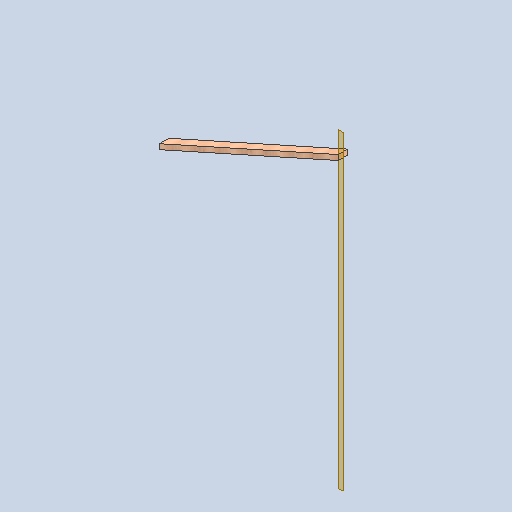
# Autodesk Inventor part: back slant
Saved by Autodesk Inventor 2025 (Build 290162000, 162)
## iProperties
Created: 2024-09-05
Part Number: back slant
Material: Wood (Birch)
Document SubType Name: Modeling
Designer: Win
Density: 0.55 g/cm^3
Appearance: Birch - Natural Polished
Author: Win
Autodesk Inventor part; units mm, degrees
ref_plane "YZ Plane" through (0, 0, 0) normal (1, 0, 0) x (0, 1, 0)
ref_plane "XZ Plane" through (0, 0, 0) normal (0, 1, 0) x (-1, 0, 0)
ref_plane "XY Plane" through (0, 0, 0) normal (0, 0, 1) x (1, 0, 0)
ref_plane "Work Plane1" through (0, 81.2927, 0) normal (0, 0, 1) x (1, 0, 0)
ref_plane "Work Plane2" through (0, 81.2927, 0) normal (0, 0, 1) x (1, 0, 0)
sketch "Sketch2" plane through (0, 81.2927, 0) normal (0, 0, 1) x (1, 0, 0)
  line L0 (-1930.4, 883.9073) -> (-1879.6, 883.9073) projected
  line L1 (-1879.6, 2103.1073) -> (-1879.6, 883.9073) projected
  line L2 (-1930.4, 2103.1073) -> (-1879.6, 2103.1073) projected
  line L3 (-1930.4, 2103.1073) -> (-1930.4, 883.9073) projected
  line L4 (-50.8, 2001.5073) -> (-50.8, 2103.1073) projected
  line L5 (-50.8, 2103.1073) -> (-1879.6, 2103.1073) projected
  line L6 (-1879.6, 2001.5073) -> (-1879.6, 2103.1073) projected
  line L7 (-50.8, 2001.5073) -> (-1879.6, 2001.5073) projected
  line L8 (0, -81.2927) -> (50.8, -81.2927) projected
  line L9 (50.8, -81.2927) -> (50.8, 2966.7073) projected
  line L10 (0, 2966.7073) -> (50.8, 2966.7073) projected
  line L11 (0, -81.2927) -> (0, 2966.7073) projected
  line L12 (-1930.4, 2103.1073) -> (0, 2966.7073)
  line L13 (0, 2966.7073) -> (0, 2911.0555)
  line L14 (-1806.0018, 2103.1073) -> (0, 2911.0555)
  line L15 (-1806.0018, 2103.1073) -> (-1930.4, 2047.4555)
  line L16 (-1930.4, 2047.4555) -> (-1930.4, 2103.1073)
  constraints: 10 end point, 3 point on line, 2 parallel, 1 collinear
extrude "Extrusion2" add sketch "Sketch2" against normal blind 101.6 contours L3 L2 L1 L15 | L12 L11 L14 L5 L2 | L1 L5 L15
body "Solid2"
